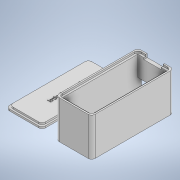
# Autodesk Inventor part: case
Saved by Autodesk Inventor 2021 (Build 250183000, 183)
## iProperties
Created: 2021-06-14
Part Number: case
Material: 일반
Document SubType Name: Modeling
Designer: dltjd
Density: 1 g/cm^3
Appearance: 기본값
Author: dltjd
Autodesk Inventor part; units mm, degrees
ref_plane "YZ Plane" through (0, 0, 0) normal (1, 0, 0) x (0, 1, 0)
ref_plane "XZ Plane" through (0, 0, 0) normal (0, 1, 0) x (-1, 0, 0)
ref_plane "XY Plane" through (0, 0, 0) normal (0, 0, 1) x (1, 0, 0)
sketch "스케치1" plane through (0, 0, 0) normal (0, 1, 0) x (-1, 0, 0)
  line L0 (14, 34) -> (-14, 34)
  line L1 (-14, 34) -> (-14, -34)
  line L2 (-14, -34) -> (14, -34)
  line L3 (14, -34) -> (14, 34)
  line L4 (14, 34) -> (-14, -34) construction
  line L5 (-14, 34) -> (14, -34) construction
  point P0 (0, 0)
  dimension "d0" = 28
  dimension "d1" = 68
  constraints: 12 end point, 2 midpoint, 2 parallel, 1 horizontal, 1 perpendicular
  measures "d0" distance of L2.end L1.end
  measures "d1" distance of L1.end L0.end
extrude "돌출1" add sketch "스케치1" along normal blind 1.5
sketch "스케치2" plane through (0, 1.5, 0) normal (0, 1, 0) x (1, 0, 0)
  line L0 (-14, 34) -> (-14, -34) projected
  line L1 (14, -34) -> (14, 34) projected
  line L2 (-14, -34) -> (14, -34)
  line L3 (14, -34) -> (14, -32.5)
  line L4 (14, -32.5) -> (-14, -32.5)
  line L5 (-14, -32.5) -> (-14, -34)
  line L6 (14, 34) -> (-14, 34) projected
  line L7 (-14, -34) -> (-12.5, -34)
  line L8 (-12.5, -34) -> (-12.5, 34)
  line L9 (-12.5, 34) -> (-14, 34)
  line L10 (-14, 34) -> (-14, -34)
  line L11 (14, -34) -> (12.5, -34)
  line L12 (12.5, -34) -> (12.5, 34)
  line L13 (12.5, 34) -> (14, 34)
  line L14 (14, 34) -> (14, -34)
  point P0 (0, 0)
  point P1 (12.5, -32.5)
  point P2 (-12.5, -32.5)
  dimension "d4" = 1.5
  dimension "d5" = 1.5
  dimension "d6" = 1.5
  constraints: 24 end point, 6 parallel, 3 horizontal, 3 perpendicular, 3 point on line
  measures "d4" distance of L3.end L2.end
  measures "d5" distance of L9.end L8.end
  measures "d6" distance of L12.end L13.end
extrude "돌출2" add sketch "스케치2" along normal blind 30 contours L6 L8 L4 L0 | L4 L8 L2 L0 | L4 L12 L2 L8 | L6 L1 L4 L12 | L4 L1 L2 L12
sketch "스케치3" plane through (0, 1.5, 0) normal (0, 1, 0) x (1, 0, 0)
  line L0 (-14, 34) -> (-14, -34) projected
  line L1 (14, -34) -> (14, 34) projected
  line L2 (-14, 34) -> (14, 34)
  line L3 (14, 34) -> (14, 32.5)
  line L4 (14, 32.5) -> (-14, 32.5)
  line L5 (-14, 32.5) -> (-14, 34)
  point P0 (0, 0)
  dimension "d9" = 1.5
  constraints: 8 end point, 2 parallel, 1 horizontal, 1 perpendicular, 1 point on line
  measures "d9" distance of L2.end L3.end
extrude "돌출3" add sketch "스케치3" along normal blind 30
sketch "스케치5" plane through (0, 1.5, 0) normal (0, 1, 0) x (1, 0, 0)
  line L0 (-27.2681, 35.5) -> (-58.2681, 35.5)
  line L1 (-58.2681, 35.5) -> (-58.2681, -35.5)
  line L2 (-58.2681, -35.5) -> (-27.2681, -35.5)
  line L3 (-27.2681, -35.5) -> (-27.2681, 35.5)
  line L4 (-27.2681, 35.5) -> (-58.2681, -35.5) construction
  line L5 (-58.2681, 35.5) -> (-27.2681, -35.5) construction
  point P0 (0, 0)
  point P1 (-42.7681, 0)
  dimension "d36" = 31
  dimension "d37" = 71
  constraints: 12 end point, 2 midpoint, 2 parallel, 1 horizontal, 1 perpendicular
  measures "d36" distance of L2.end L1.end
  measures "d37" distance of L1.end L0.end
ref_plane "작업 평면1" through (0, 3, 0) normal (0, 1, 0) x (1, 0, 0)
sketch "스케치7" plane through (14, 0, -34) normal (0, 0, -1) x (-1, 0, 0)
  line L0 (0, 31.5) -> (28, 31.5) projected
  line L1 (0, 31.5) -> (28, 31.5)
  line L2 (28, 31.5) -> (28, 0)
  line L3 (28, 0) -> (0, 0)
  line L4 (0, 0) -> (0, 31.5)
  point P0 (14, 0)
  constraints: 8 end point, 2 parallel, 1 horizontal, 1 perpendicular
extrude "돌출7" add sketch "스케치7" along normal blind 1.5
sketch "스케치8" plane through (0, 1.5, 0) normal (0, 1, 0) x (1, 0, 0)
  line L0 (12.5, 32.5) -> (12.5, -32.5) projected
  line L1 (14, 35.5) -> (-14, 35.5) projected
  line L2 (12.5, 32.5) -> (-12.5, 32.5)
  line L3 (-12.5, 32.5) -> (-12.5, 35.5)
  line L4 (-12.5, 35.5) -> (12.5, 35.5)
  line L5 (12.5, 35.5) -> (12.5, 32.5)
  point P0 (0, 0)
  dimension "d26" = 25
  constraints: 8 end point, 2 parallel, 1 horizontal, 1 perpendicular, 1 point on line
  measures "d26" distance of L3.end L4.end
sketch "스케치9" plane through (14, 0, 34) normal (1, 0, 0) x (0, 0, -1)
  line L0 (0, 31.5) -> (69.5, 31.5) projected
  line L1 (69.5, 31.5) -> (0, 31.5)
  line L2 (0, 31.5) -> (0, 0)
  line L3 (0, 0) -> (69.5, 0)
  line L4 (69.5, 0) -> (69.5, 31.5)
  point P0 (34, 0)
  constraints: 8 end point, 2 parallel, 1 horizontal, 1 perpendicular
extrude "돌출9" add sketch "스케치9" along normal blind 1.5
sketch "스케치10" plane through (-14, 0, 34) normal (0, 0, 1) x (1, 0, 0)
  line L0 (0, 0) -> (0, 31.5) projected
  line L1 (29.5, 31.5) -> (29.5, 0) projected
  line L2 (0, 31.5) -> (29.5, 31.5)
  line L3 (29.5, 31.5) -> (29.5, 0)
  line L4 (29.5, 0) -> (0, 0)
  line L5 (0, 0) -> (0, 31.5)
  point P0 (14, 0)
  constraints: 8 end point, 2 parallel, 1 horizontal, 1 perpendicular
extrude "돌출10" add sketch "스케치10" along normal blind 1.5
sketch "스케치11" plane through (-14, 0, -35.5) normal (-1, 0, 0) x (0, 0, 1)
  line L0 (0, 31.5) -> (71, 31.5) projected
  line L1 (0, 0) -> (71, 0)
  line L2 (71, 0) -> (71, 31.5)
  line L3 (71, 31.5) -> (0, 31.5)
  line L4 (0, 31.5) -> (0, 0)
  point P0 (35.5, 0)
  constraints: 8 end point, 2 parallel, 1 horizontal, 1 perpendicular
extrude "돌출11" add sketch "스케치11" along normal blind 1.5
fillet "모깎기1" radius 3 4 edges at (15.5, 15.75, -35.5) (-15.5, 15.75, -35.5) (-15.5, 15.75, 35.5) (15.5, 15.75, 35.5)
extrude "돌출12" add sketch "스케치5" along normal blind 1.5
fillet "모깎기2" radius 3 4 edges at (-58.2681, 2.25, 35.5) (-27.2681, 2.25, 35.5) (-27.2681, 2.25, -35.5) (-58.2681, 2.25, -35.5)
sketch "스케치12" plane through (0, 31.5, 0) normal (0, 1, 0) x (1, 0, 0)
  line L0 (-14, -31.6724) -> (-14, -27.7757)
  line L1 (14, 29.0808) -> (14, 30.2026)
  line L2 (-12.5, 32.5) -> (12.5, 32.5) projected
  line L3 (7.6672, 32.5) -> (14, 32.5)
  line L4 (-11, -34) -> (11, -34)
  line L5 (14, -31) -> (14, 31)
  line L6 (11, 34) -> (-11, 34)
  line L7 (-14, 31) -> (-14, -31)
  line L8 (-12.5, -35.5) -> (12.5, -35.5)
  line L9 (15.5, -32.5) -> (15.5, 32.5)
  line L10 (12.5, 35.5) -> (-12.5, 35.5)
  line L11 (-15.5, 32.5) -> (-15.5, -32.5)
  arc A0 (-15.5, -32.5) -> (-12.5, -35.5) centre (-12.5, -32.5) ccw
  arc A1 (12.5, -35.5) -> (15.5, -32.5) centre (12.5, -32.5) ccw
  arc A2 (15.5, 32.5) -> (12.5, 35.5) centre (12.5, 32.5) ccw
  arc A3 (-12.5, 35.5) -> (-15.5, 32.5) centre (-12.5, 32.5) ccw
  arc A4 (14, 31) -> (11, 34) centre (11, 31) ccw
  arc A5 (-11, 34) -> (-14, 31) centre (-11, 31) ccw
  arc A6 (-14, -31) -> (-11, -34) centre (-11, -31) ccw
  arc A7 (11, -34) -> (14, -31) centre (11, -31) ccw
  point P0 (0, 0)
  dimension "d45" = 3
  constraints: 22 end point, 16 point on circle, 16 tangent, 8 centre point, 7 equal radius, 4 parallel, 3 horizontal, 2 perpendicular, 1 point on line
  measures "d45" radius of A0
extrude "돌출13" add sketch "스케치12" along normal blind 1.5
sketch "스케치13" plane through (0, 3, 0) normal (0, 1, 0) x (1, 0, 0)
  line L0 (-58.2681, 32.5) -> (-58.2681, -32.5) projected
  line L1 (-55.2681, -35.5) -> (-30.2681, -35.5) projected
  line L2 (-27.2681, -32.5) -> (-27.2681, 32.5) projected
  line L3 (-30.2681, 35.5) -> (-55.2681, 35.5) projected
  line L4 (-53.7681, -34) -> (-31.7681, -34)
  line L5 (-28.7681, -31) -> (-28.7681, 31)
  line L6 (-31.7681, 34) -> (-53.7681, 34)
  line L7 (-56.7681, 31) -> (-56.7681, -31)
  arc A0 (-56.7681, -31) -> (-53.7681, -34) centre (-53.7681, -31) ccw
  arc A1 (-31.7681, -34) -> (-28.7681, -31) centre (-31.7681, -31) ccw
  arc A2 (-28.7681, 31) -> (-31.7681, 34) centre (-31.7681, 31) ccw
  arc A3 (-53.7681, 34) -> (-56.7681, 31) centre (-53.7681, 31) ccw
  point P0 (0, 0)
  point P1 (-56.7681, -34)
  point P2 (-28.7681, 34)
  dimension "d54" = 3
  constraints: 8 end point, 8 point on circle, 8 tangent, 4 centre point, 4 point on line, 3 equal radius, 2 parallel, 1 horizontal, 1 perpendicular
  measures "d54" radius of A0
extrude "돌출15" add sketch "스케치13" along normal blind 1.5
sketch "스케치14" plane through (0, 1.5, 0) normal (0, -1, 0) x (1, 0, 0)
  line L0 (-44.3921, -14.3977) -> (-44.3921, 14.3977) construction
  line L1 (-44.3921, 14.3977) -> (-41.144, 14.3977) construction
  line L2 (-41.144, 14.3977) -> (-41.144, -14.3977) construction
  line L3 (-41.144, -14.3977) -> (-44.3921, -14.3977) construction
  line L4 (-30.2681, -35.5) -> (-55.2681, -35.5) projected
  line L5 (-58.2681, -32.5) -> (-58.2681, 32.5) projected
  line L6 (-41.2083, -11.7301) -> (-41.2083, -12.2562)
  line L7 (-41.2083, -12.2562) -> (-42.421, -13.2195)
  line L8 (-42.421, -13.2195) -> (-42.421, -13.6839)
  line L9 (-42.421, -13.6839) -> (-41.2083, -13.6839)
  line L10 (-41.2083, -13.6839) -> (-41.2083, -14.089)
  line L11 (-41.2083, -14.089) -> (-44.2563, -14.089)
  line L12 (-44.2563, -14.089) -> (-44.2563, -13.3035)
  spline S0 degree 2 poles (-44.2563, -13.3035) (-44.2563, -13.0417) (-44.1995, -12.6885) (-44.0957, -12.5279) knots 0 0 0 1 2 2 2
  spline S1 degree 2 poles (-44.0957, -12.5279) (-43.992, -12.3674) (-43.6684, -12.1821) (-43.4288, -12.1821) knots 0 0 0 1 2 2 2
  spline S2 degree 2 poles (-43.4288, -12.1821) (-43.0954, -12.1821) (-42.6433, -12.523) (-42.5347, -12.8144) knots 0 0 0 1 2 2 2
  line L13 (-42.5347, -12.8144) -> (-41.2083, -11.7301)
  spline S3 degree 2 poles (-43.3967, -12.6045) (-43.5301, -12.6045) (-43.7351, -12.6984) (-43.8018, -12.7972) knots 0 0 0 1 2 2 2
  spline S4 degree 2 poles (-43.8018, -12.7972) (-43.8586, -12.8836) (-43.9055, -13.1133) (-43.9055, -13.2813) knots 0 0 0 1 2 2 2
  line L14 (-43.9055, -13.2813) -> (-43.9055, -13.6839)
  line L15 (-43.9055, -13.6839) -> (-42.7594, -13.6839)
  line L16 (-42.7594, -13.6839) -> (-42.7594, -13.3282)
  spline S5 degree 2 poles (-42.7594, -13.3282) (-42.7594, -13.1528) (-42.8212, -12.8737) (-42.9175, -12.7774) knots 0 0 0 1 2 2 2
  spline S6 degree 2 poles (-42.9175, -12.7774) (-43.0015, -12.6885) (-43.2386, -12.6045) (-43.3967, -12.6045) knots 0 0 0 1 2 2 2
  spline S7 degree 2 poles (-41.1564, -10.5247) (-41.1564, -11.0731) (-41.7714, -11.6758) (-42.3395, -11.6758) knots 0 0 0 1 2 2 2
  spline S8 degree 2 poles (-42.3395, -11.6758) (-42.8978, -11.6758) (-43.5597, -11.0904) (-43.5597, -10.6186) knots 0 0 0 1 2 2 2
  spline S9 degree 2 poles (-43.5597, -10.6186) (-43.5597, -10.4062) (-43.4362, -10.0777) (-43.3053, -9.9566) knots 0 0 0 1 2 2 2
  spline S10 degree 2 poles (-43.3053, -9.9566) (-43.1744, -9.8331) (-42.7965, -9.7022) (-42.5223, -9.7022) knots 0 0 0 1 2 2 2
  line L17 (-42.5223, -9.7022) -> (-42.3124, -9.7022)
  line L18 (-42.3124, -9.7022) -> (-42.3124, -11.2855)
  spline S11 degree 2 poles (-42.3124, -11.2855) (-41.9147, -11.2855) (-41.4923, -10.8854) (-41.4923, -10.5297) knots 0 0 0 1 2 2 2
  spline S12 degree 2 poles (-41.4923, -10.5297) (-41.4923, -10.4037) (-41.5491, -10.1592) (-41.5936, -10.0604) knots 0 0 0 1 2 2 2
  spline S13 degree 2 poles (-41.5936, -10.0604) (-41.643, -9.9566) (-41.7294, -9.8134) (-41.769, -9.7664) knots 0 0 0 1 2 2 2
  line L19 (-41.769, -9.7664) -> (-41.769, -9.7442)
  line L20 (-41.769, -9.7442) -> (-41.3491, -9.7442)
  spline S14 degree 2 poles (-41.3491, -9.7442) (-41.3219, -9.8109) (-41.2428, -10.0134) (-41.2206, -10.0925) knots 0 0 0 1 2 2 2
  spline S15 degree 2 poles (-41.2206, -10.0925) (-41.1885, -10.2036) (-41.1564, -10.3864) (-41.1564, -10.5247) knots 0 0 0 1 2 2 2
  spline S16 degree 2 poles (-42.6063, -10.0777) (-42.7619, -10.0826) (-42.9891, -10.1468) (-43.0657, -10.2086) knots 0 0 0 1 2 2 2
  spline S17 degree 2 poles (-43.0657, -10.2086) (-43.1522, -10.2753) (-43.2436, -10.4852) (-43.2436, -10.6408) knots 0 0 0 1 2 2 2
  spline S18 degree 2 poles (-43.2436, -10.6408) (-43.2436, -10.794) (-43.1522, -11.0089) (-43.0632, -11.0978) knots 0 0 0 1 2 2 2
  spline S19 degree 2 poles (-43.0632, -11.0978) (-42.9719, -11.1842) (-42.752, -11.2732) (-42.6063, -11.2855) knots 0 0 0 1 2 2 2
  line L21 (-42.6063, -11.2855) -> (-42.6063, -10.0777)
  line L22 (-41.2083, -6.7184) -> (-42.5322, -6.7184)
  spline S20 degree 2 poles (-42.5322, -6.7184) (-42.6903, -6.7184) (-42.9595, -6.7431) (-43.0336, -6.7827) knots 0 0 0 1 2 2 2
  spline S21 degree 2 poles (-43.0336, -6.7827) (-43.1151, -6.8222) (-43.1942, -6.9729) (-43.1942, -7.1038) knots 0 0 0 1 2 2 2
  spline S22 degree 2 poles (-43.1942, -7.1038) (-43.1942, -7.2223) (-43.0484, -7.494) (-42.9101, -7.6373) knots 0 0 0 1 2 2 2
  spline S23 degree 2 poles (-42.9101, -7.6373) (-42.8755, -7.6348) (-42.7792, -7.6299) (-42.715, -7.6299) knots 0 0 0 1 2 2 2
  line L23 (-42.715, -7.6299) -> (-41.2083, -7.6299)
  line L24 (-41.2083, -7.6299) -> (-41.2083, -8.0152)
  line L25 (-41.2083, -8.0152) -> (-42.5322, -8.0152)
  spline S24 degree 2 poles (-42.5322, -8.0152) (-42.6903, -8.0152) (-42.9595, -8.0399) (-43.0336, -8.0794) knots 0 0 0 1 2 2 2
  spline S25 degree 2 poles (-43.0336, -8.0794) (-43.1151, -8.1189) (-43.1942, -8.2696) (-43.1942, -8.4005) knots 0 0 0 1 2 2 2
  spline S26 degree 2 poles (-43.1942, -8.4005) (-43.1942, -8.524) (-43.0385, -8.7982) (-42.9175, -8.9266) knots 0 0 0 1 2 2 2
  line L26 (-42.9175, -8.9266) -> (-41.2083, -8.9266)
  line L27 (-41.2083, -8.9266) -> (-41.2083, -9.312)
  line L28 (-41.2083, -9.312) -> (-43.4955, -9.312)
  line L29 (-43.4955, -9.312) -> (-43.4955, -8.9266)
  line L30 (-43.4955, -8.9266) -> (-43.2436, -8.9266)
  spline S27 degree 2 poles (-43.2436, -8.9266) (-43.3942, -8.776) (-43.5597, -8.4796) (-43.5597, -8.3017) knots 0 0 0 1 2 2 2
  spline S28 degree 2 poles (-43.5597, -8.3017) (-43.5597, -8.0992) (-43.3745, -7.7855) (-43.1645, -7.704) knots 0 0 0 1 2 2 2
  spline S29 degree 2 poles (-43.1645, -7.704) (-43.3596, -7.5286) (-43.5597, -7.1976) (-43.5597, -7.005) knots 0 0 0 1 2 2 2
  spline S30 degree 2 poles (-43.5597, -7.005) (-43.5597, -6.8568) (-43.4683, -6.6147) (-43.3646, -6.5258) knots 0 0 0 1 2 2 2
  spline S31 degree 2 poles (-43.3646, -6.5258) (-43.2608, -6.4344) (-42.9496, -6.3331) (-42.715, -6.3331) knots 0 0 0 1 2 2 2
  line L31 (-42.715, -6.3331) -> (-41.2083, -6.3331)
  line L32 (-41.2083, -6.3331) -> (-41.2083, -6.7184)
  spline S32 degree 2 poles (-42.3519, -3.9125) (-41.7739, -3.9125) (-41.144, -4.4683) (-41.144, -4.9326) knots 0 0 0 1 2 2 2
  spline S33 degree 2 poles (-41.144, -4.9326) (-41.144, -5.4093) (-41.7937, -5.9552) (-42.3519, -5.9552) knots 0 0 0 1 2 2 2
  spline S34 degree 2 poles (-42.3519, -5.9552) (-42.9249, -5.9552) (-43.5597, -5.392) (-43.5597, -4.9326) knots 0 0 0 1 2 2 2
  spline S35 degree 2 poles (-43.5597, -4.9326) (-43.5597, -4.4683) (-42.9274, -3.9125) (-42.3519, -3.9125) knots 0 0 0 1 2 2 2
  spline S36 degree 2 poles (-42.3519, -4.3102) (-42.7965, -4.3102) (-43.2287, -4.6338) (-43.2287, -4.9326) knots 0 0 0 1 2 2 2
  spline S37 degree 2 poles (-43.2287, -4.9326) (-43.2287, -5.2315) (-42.7965, -5.5575) (-42.3519, -5.5575) knots 0 0 0 1 2 2 2
  spline S38 degree 2 poles (-42.3519, -5.5575) (-41.9196, -5.5575) (-41.475, -5.2315) (-41.475, -4.9326) knots 0 0 0 1 2 2 2
  spline S39 degree 2 poles (-41.475, -4.9326) (-41.475, -4.6362) (-41.9122, -4.3102) (-42.3519, -4.3102) knots 0 0 0 1 2 2 2
  spline S40 degree 2 poles (-41.1638, -2.8257) (-41.1638, -3.1394) (-41.522, -3.4926) (-41.9098, -3.4926) knots 0 0 0 1 2 2 2
  line L33 (-41.9098, -3.4926) -> (-43.1769, -3.4926)
  line L34 (-43.1769, -3.4926) -> (-43.1769, -3.752)
  line L35 (-43.1769, -3.752) -> (-43.4955, -3.752)
  line L36 (-43.4955, -3.752) -> (-43.4955, -3.4926)
  line L37 (-43.4955, -3.4926) -> (-44.1525, -3.4926)
  line L38 (-44.1525, -3.4926) -> (-44.1525, -3.1073)
  line L39 (-44.1525, -3.1073) -> (-43.4955, -3.1073)
  line L40 (-43.4955, -3.1073) -> (-43.4955, -2.3984)
  line L41 (-43.4955, -2.3984) -> (-43.1769, -2.3984)
  line L42 (-43.1769, -2.3984) -> (-43.1769, -3.1073)
  line L43 (-43.1769, -3.1073) -> (-42.0876, -3.1073)
  spline S41 degree 2 poles (-42.0876, -3.1073) (-41.9147, -3.1073) (-41.7245, -3.0949) (-41.643, -3.0529) knots 0 0 0 1 2 2 2
  spline S42 degree 2 poles (-41.643, -3.0529) (-41.5714, -3.0184) (-41.4997, -2.8627) (-41.4997, -2.7294) knots 0 0 0 1 2 2 2
  spline S43 degree 2 poles (-41.4997, -2.7294) (-41.4997, -2.6355) (-41.5565, -2.4601) (-41.5738, -2.4206) knots 0 0 0 1 2 2 2
  line L44 (-41.5738, -2.4206) -> (-41.5738, -2.3984)
  line L45 (-41.5738, -2.3984) -> (-41.228, -2.3984)
  spline S44 degree 2 poles (-41.228, -2.3984) (-41.1984, -2.5071) (-41.1638, -2.7294) (-41.1638, -2.8257) knots 0 0 0 1 2 2 2
  spline S45 degree 2 poles (-41.1564, -1.1214) (-41.1564, -1.6697) (-41.7714, -2.2724) (-42.3395, -2.2724) knots 0 0 0 1 2 2 2
  spline S46 degree 2 poles (-42.3395, -2.2724) (-42.8978, -2.2724) (-43.5597, -1.687) (-43.5597, -1.2152) knots 0 0 0 1 2 2 2
  spline S47 degree 2 poles (-43.5597, -1.2152) (-43.5597, -1.0028) (-43.4362, -0.6743) (-43.3053, -0.5533) knots 0 0 0 1 2 2 2
  spline S48 degree 2 poles (-43.3053, -0.5533) (-43.1744, -0.4298) (-42.7965, -0.2989) (-42.5223, -0.2989) knots 0 0 0 1 2 2 2
  line L46 (-42.5223, -0.2989) -> (-42.3124, -0.2989)
  line L47 (-42.3124, -0.2989) -> (-42.3124, -1.8822)
  spline S49 degree 2 poles (-42.3124, -1.8822) (-41.9147, -1.8822) (-41.4923, -1.482) (-41.4923, -1.1263) knots 0 0 0 1 2 2 2
  spline S50 degree 2 poles (-41.4923, -1.1263) (-41.4923, -1.0004) (-41.5491, -0.7558) (-41.5936, -0.657) knots 0 0 0 1 2 2 2
  spline S51 degree 2 poles (-41.5936, -0.657) (-41.643, -0.5533) (-41.7294, -0.41) (-41.769, -0.3631) knots 0 0 0 1 2 2 2
  line L48 (-41.769, -0.3631) -> (-41.769, -0.3409)
  line L49 (-41.769, -0.3409) -> (-41.3491, -0.3409)
  spline S52 degree 2 poles (-41.3491, -0.3409) (-41.3219, -0.4076) (-41.2428, -0.6101) (-41.2206, -0.6891) knots 0 0 0 1 2 2 2
  spline S53 degree 2 poles (-41.2206, -0.6891) (-41.1885, -0.8003) (-41.1564, -0.9831) (-41.1564, -1.1214) knots 0 0 0 1 2 2 2
  spline S54 degree 2 poles (-42.6063, -0.6743) (-42.7619, -0.6793) (-42.9891, -0.7435) (-43.0657, -0.8052) knots 0 0 0 1 2 2 2
  spline S55 degree 2 poles (-43.0657, -0.8052) (-43.1522, -0.8719) (-43.2436, -1.0819) (-43.2436, -1.2375) knots 0 0 0 1 2 2 2
  spline S56 degree 2 poles (-43.2436, -1.2375) (-43.2436, -1.3906) (-43.1522, -1.6055) (-43.0632, -1.6944) knots 0 0 0 1 2 2 2
  spline S57 degree 2 poles (-43.0632, -1.6944) (-42.9719, -1.7809) (-42.752, -1.8698) (-42.6063, -1.8822) knots 0 0 0 1 2 2 2
  line L50 (-42.6063, -1.8822) -> (-42.6063, -0.6743)
  spline S58 degree 2 poles (-41.1539, 2.6207) (-41.1539, 2.3243) (-41.354, 1.8229) (-41.5541, 1.6401) knots 0 0 0 1 2 2 2
  spline S59 degree 2 poles (-41.5541, 1.6401) (-41.7517, 1.4573) (-42.3445, 1.2572) (-42.7298, 1.2572) knots 0 0 0 1 2 2 2
  spline S60 degree 2 poles (-42.7298, 1.2572) (-43.1126, 1.2572) (-43.6808, 1.4524) (-43.8907, 1.6376) knots 0 0 0 1 2 2 2
  spline S61 degree 2 poles (-43.8907, 1.6376) (-44.0957, 1.8204) (-44.3106, 2.3193) (-44.3106, 2.6281) knots 0 0 0 1 2 2 2
  spline S62 degree 2 poles (-44.3106, 2.6281) (-44.3106, 2.7812) (-44.2661, 3.0505) (-44.2316, 3.1641) knots 0 0 0 1 2 2 2
  spline S63 degree 2 poles (-44.2316, 3.1641) (-44.1995, 3.2629) (-44.1081, 3.4679) (-44.0537, 3.5692) knots 0 0 0 1 2 2 2
  line L51 (-44.0537, 3.5692) -> (-43.5647, 3.5692)
  line L52 (-43.5647, 3.5692) -> (-43.5647, 3.5371)
  spline S64 degree 2 poles (-43.5647, 3.5371) (-43.6141, 3.4827) (-43.7524, 3.3148) (-43.8191, 3.1937) knots 0 0 0 1 2 2 2
  spline S65 degree 2 poles (-43.8191, 3.1937) (-43.8833, 3.0776) (-43.9648, 2.8035) (-43.9648, 2.6256) knots 0 0 0 1 2 2 2
  spline S66 degree 2 poles (-43.9648, 2.6256) (-43.9648, 2.4305) (-43.8043, 2.0822) (-43.6511, 1.9513) knots 0 0 0 1 2 2 2
  spline S67 degree 2 poles (-43.6511, 1.9513) (-43.4955, 1.8229) (-43.0237, 1.6796) (-42.7298, 1.6796) knots 0 0 0 1 2 2 2
  spline S68 degree 2 poles (-42.7298, 1.6796) (-42.4161, 1.6796) (-41.9641, 1.8303) (-41.8085, 1.9612) knots 0 0 0 1 2 2 2
  spline S69 degree 2 poles (-41.8085, 1.9612) (-41.6578, 2.0896) (-41.5047, 2.433) (-41.5047, 2.6256) knots 0 0 0 1 2 2 2
  spline S70 degree 2 poles (-41.5047, 2.6256) (-41.5047, 2.801) (-41.5911, 3.0999) (-41.6553, 3.216) knots 0 0 0 1 2 2 2
  spline S71 degree 2 poles (-41.6553, 3.216) (-41.7196, 3.3271) (-41.8529, 3.4926) (-41.8999, 3.5395) knots 0 0 0 1 2 2 2
  line L53 (-41.8999, 3.5395) -> (-41.8999, 3.5692)
  line L54 (-41.8999, 3.5692) -> (-41.4157, 3.5692)
  spline S72 degree 2 poles (-41.4157, 3.5692) (-41.3688, 3.4679) (-41.2824, 3.2901) (-41.2428, 3.1641) knots 0 0 0 1 2 2 2
  spline S73 degree 2 poles (-41.2428, 3.1641) (-41.1984, 3.0307) (-41.1539, 2.8035) (-41.1539, 2.6207) knots 0 0 0 1 2 2 2
  spline S74 degree 2 poles (-42.3519, 5.7971) (-41.7739, 5.7971) (-41.144, 5.2414) (-41.144, 4.777) knots 0 0 0 1 2 2 2
  spline S75 degree 2 poles (-41.144, 4.777) (-41.144, 4.3003) (-41.7937, 3.7544) (-42.3519, 3.7544) knots 0 0 0 1 2 2 2
  spline S76 degree 2 poles (-42.3519, 3.7544) (-42.9249, 3.7544) (-43.5597, 4.3176) (-43.5597, 4.777) knots 0 0 0 1 2 2 2
  spline S77 degree 2 poles (-43.5597, 4.777) (-43.5597, 5.2414) (-42.9274, 5.7971) (-42.3519, 5.7971) knots 0 0 0 1 2 2 2
  spline S78 degree 2 poles (-42.3519, 5.3995) (-42.7965, 5.3995) (-43.2287, 5.0759) (-43.2287, 4.777) knots 0 0 0 1 2 2 2
  spline S79 degree 2 poles (-43.2287, 4.777) (-43.2287, 4.4781) (-42.7965, 4.1521) (-42.3519, 4.1521) knots 0 0 0 1 2 2 2
  spline S80 degree 2 poles (-42.3519, 4.1521) (-41.9196, 4.1521) (-41.475, 4.4781) (-41.475, 4.777) knots 0 0 0 1 2 2 2
  spline S81 degree 2 poles (-41.475, 4.777) (-41.475, 5.0734) (-41.9122, 5.3995) (-42.3519, 5.3995) knots 0 0 0 1 2 2 2
  line L55 (-41.2083, 7.988) -> (-41.2083, 7.6027)
  line L56 (-41.2083, 7.6027) -> (-42.5124, 7.6027)
  spline S82 degree 2 poles (-42.5124, 7.6027) (-42.6705, 7.6027) (-42.9422, 7.5731) (-43.0237, 7.5286) knots 0 0 0 1 2 2 2
  spline S83 degree 2 poles (-43.0237, 7.5286) (-43.1102, 7.4817) (-43.1942, 7.3137) (-43.1942, 7.1705) knots 0 0 0 1 2 2 2
  spline S84 degree 2 poles (-43.1942, 7.1705) (-43.1942, 7.0272) (-43.041, 6.7234) (-42.9175, 6.5777) knots 0 0 0 1 2 2 2
  line L57 (-42.9175, 6.5777) -> (-41.2083, 6.5777)
  line L58 (-41.2083, 6.5777) -> (-41.2083, 6.1923)
  line L59 (-41.2083, 6.1923) -> (-43.4955, 6.1923)
  line L60 (-43.4955, 6.1923) -> (-43.4955, 6.5777)
  line L61 (-43.4955, 6.5777) -> (-43.2411, 6.5777)
  spline S85 degree 2 poles (-43.2411, 6.5777) (-43.3967, 6.7506) (-43.5597, 7.084) (-43.5597, 7.2717) knots 0 0 0 1 2 2 2
  spline S86 degree 2 poles (-43.5597, 7.2717) (-43.5597, 7.6076) (-43.1151, 7.988) (-42.6927, 7.988) knots 0 0 0 1 2 2 2
  line L62 (-42.6927, 7.988) -> (-41.2083, 7.988)
  spline S87 degree 2 poles (-41.1638, 9.2206) (-41.1638, 8.9069) (-41.522, 8.5537) (-41.9098, 8.5537) knots 0 0 0 1 2 2 2
  line L63 (-41.9098, 8.5537) -> (-43.1769, 8.5537)
  line L64 (-43.1769, 8.5537) -> (-43.1769, 8.2943)
  line L65 (-43.1769, 8.2943) -> (-43.4955, 8.2943)
  line L66 (-43.4955, 8.2943) -> (-43.4955, 8.5537)
  line L67 (-43.4955, 8.5537) -> (-44.1525, 8.5537)
  line L68 (-44.1525, 8.5537) -> (-44.1525, 8.939)
  line L69 (-44.1525, 8.939) -> (-43.4955, 8.939)
  line L70 (-43.4955, 8.939) -> (-43.4955, 9.6479)
  line L71 (-43.4955, 9.6479) -> (-43.1769, 9.6479)
  line L72 (-43.1769, 9.6479) -> (-43.1769, 8.939)
  line L73 (-43.1769, 8.939) -> (-42.0876, 8.939)
  spline S88 degree 2 poles (-42.0876, 8.939) (-41.9147, 8.939) (-41.7245, 8.9513) (-41.643, 8.9933) knots 0 0 0 1 2 2 2
  spline S89 degree 2 poles (-41.643, 8.9933) (-41.5714, 9.0279) (-41.4997, 9.1835) (-41.4997, 9.3169) knots 0 0 0 1 2 2 2
  spline S90 degree 2 poles (-41.4997, 9.3169) (-41.4997, 9.4108) (-41.5565, 9.5861) (-41.5738, 9.6257) knots 0 0 0 1 2 2 2
  line L74 (-41.5738, 9.6257) -> (-41.5738, 9.6479)
  line L75 (-41.5738, 9.6479) -> (-41.228, 9.6479)
  spline S91 degree 2 poles (-41.228, 9.6479) (-41.1984, 9.5392) (-41.1638, 9.3169) (-41.1638, 9.2206) knots 0 0 0 1 2 2 2
  line L76 (-43.083, 11.1447) -> (-43.083, 11.125)
  spline S92 degree 2 poles (-43.083, 11.125) (-43.0954, 11.0805) (-43.1003, 10.9842) (-43.1003, 10.9175) knots 0 0 0 1 2 2 2
  spline S93 degree 2 poles (-43.1003, 10.9175) (-43.1003, 10.7619) (-42.9644, 10.4556) (-42.8311, 10.3173) knots 0 0 0 1 2 2 2
  line L77 (-42.8311, 10.3173) -> (-41.2083, 10.3173)
  line L78 (-41.2083, 10.3173) -> (-41.2083, 9.9319)
  line L79 (-41.2083, 9.9319) -> (-43.4955, 9.9319)
  line L80 (-43.4955, 9.9319) -> (-43.4955, 10.3173)
  line L81 (-43.4955, 10.3173) -> (-43.1546, 10.3173)
  spline S94 degree 2 poles (-43.1546, 10.3173) (-43.3424, 10.5272) (-43.4955, 10.8409) (-43.4955, 10.9891) knots 0 0 0 1 2 2 2
  spline S95 degree 2 poles (-43.4955, 10.9891) (-43.4955, 11.0484) (-43.4906, 11.1077) (-43.4832, 11.1447) knots 0 0 0 1 2 2 2
  line L82 (-43.4832, 11.1447) -> (-43.083, 11.1447)
  spline S96 degree 2 poles (-42.3519, 13.3233) (-41.7739, 13.3233) (-41.144, 12.7675) (-41.144, 12.3032) knots 0 0 0 1 2 2 2
  spline S97 degree 2 poles (-41.144, 12.3032) (-41.144, 11.8264) (-41.7937, 11.2806) (-42.3519, 11.2806) knots 0 0 0 1 2 2 2
  spline S98 degree 2 poles (-42.3519, 11.2806) (-42.9249, 11.2806) (-43.5597, 11.8437) (-43.5597, 12.3032) knots 0 0 0 1 2 2 2
  spline S99 degree 2 poles (-43.5597, 12.3032) (-43.5597, 12.7675) (-42.9274, 13.3233) (-42.3519, 13.3233) knots 0 0 0 1 2 2 2
  spline S100 degree 2 poles (-42.3519, 12.9256) (-42.7965, 12.9256) (-43.2287, 12.602) (-43.2287, 12.3032) knots 0 0 0 1 2 2 2
  spline S101 degree 2 poles (-43.2287, 12.3032) (-43.2287, 12.0043) (-42.7965, 11.6782) (-42.3519, 11.6782) knots 0 0 0 1 2 2 2
  spline S102 degree 2 poles (-42.3519, 11.6782) (-41.9196, 11.6782) (-41.475, 12.0043) (-41.475, 12.3032) knots 0 0 0 1 2 2 2
  spline S103 degree 2 poles (-41.475, 12.3032) (-41.475, 12.5996) (-41.9122, 12.9256) (-42.3519, 12.9256) knots 0 0 0 1 2 2 2
  line L83 (-41.2083, 14.1112) -> (-41.2083, 13.7259)
  line L84 (-41.2083, 13.7259) -> (-44.3921, 13.7259)
  line L85 (-44.3921, 13.7259) -> (-44.3921, 14.1112)
  line L86 (-44.3921, 14.1112) -> (-41.2083, 14.1112)
  point P0 (0, 0)
  point P1 (-42.7681, -14.3977)
  point P2 (-42.7681, -35.5)
  point P3 (-58.2681, 0)
  point P4 (-44.3921, 0)
  constraints: 4 midpoint, 1 horizontal alignment, 1 vertical alignment, 2 other
extrude "돌출16" cut sketch "스케치14" against normal blind 10
sketch "스케치15" plane through (14, 0, -35.5) normal (0, 0, -1) x (-1, 0, 0)
  line L0 (26.5, 33) -> (1.5, 33) projected
  line L1 (6.5, 30) -> (21.5, 30)
  line L2 (21.5, 30) -> (21.5, 33)
  line L3 (21.5, 33) -> (6.5, 33)
  line L4 (6.5, 33) -> (6.5, 30)
  line L5 (1.5, 31.5) -> (26.5, 31.5) projected
  line L6 (6.5, 30) -> (21.5, 33) construction
  line L7 (21.5, 30) -> (6.5, 33) construction
  point P0 (14, 0)
  point P1 (14, 31.5)
  dimension "d59" = 15
  constraints: 12 end point, 3 midpoint, 2 parallel, 1 horizontal, 1 perpendicular, 1 point on line
  measures "d59" distance of L3.end L2.end
extrude "돌출17" cut sketch "스케치15" against normal blind 10
extrude "돌출18" cut sketch "스케치8" along normal blind 12.5
sketch "스케치16" plane through (0, 33, 0) normal (0, 1, 0) x (1, 0, 0)
  line L0 (-11.25, -34.25) -> (11.25, -34.25)
  line L1 (14.25, -31.25) -> (14.25, 31.25)
  line L2 (11.25, 34.25) -> (-11.25, 34.25)
  line L3 (-14.25, 31.25) -> (-14.25, -31.25)
  line L4 (-14.25, -34.25) -> (14.25, 34.25) construction
  line L5 (14.25, -34.25) -> (-14.25, 34.25) construction
  arc A0 (-14.25, -31.25) -> (-11.25, -34.25) centre (-11.25, -31.25) ccw
  arc A1 (11.25, -34.25) -> (14.25, -31.25) centre (11.25, -31.25) ccw
  arc A2 (14.25, 31.25) -> (11.25, 34.25) centre (11.25, 31.25) ccw
  arc A3 (-11.25, 34.25) -> (-14.25, 31.25) centre (-11.25, 31.25) ccw
  point P0 (0, 0)
  dimension "d64" = 28.5
  dimension "d65" = 68.5
  dimension "d66" = 3
  constraints: 12 end point, 8 point on circle, 8 point on line, 8 tangent, 4 centre point, 3 equal radius, 2 midpoint, 2 parallel, 1 horizontal, 1 perpendicular
  measures "d64" distance of L5.end L4.end
  measures "d65" distance of L4.end L5.start
  measures "d66" radius of A0
extrude "돌출19" cut sketch "스케치16" against normal blind 1.5
sketch "스케치17" plane through (0, 3, 0) normal (0, 1, 0) x (1, 0, 0)
  point P0 (0, 0)
